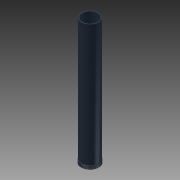
# Autodesk Inventor part: 13_0204_027
Saved by Autodesk Inventor 2012 SP1 (Build 160190100, 190)
## iProperties
Created: 2013-04-03
Part Number: 13_0204_027
Material: Default
Document SubType Name: Modeling
Designer: vogel
Density: 1 g/cm^3
Author: vogel
Autodesk Inventor part; units mm, degrees
ref_plane "YZ Plane" through (0, 0, 0) normal (1, 0, 0) x (0, 1, 0)
ref_plane "XZ Plane" through (0, 0, 0) normal (0, 1, 0) x (-1, 0, 0)
ref_plane "XY Plane" through (0, 0, 0) normal (0, 0, 1) x (1, 0, 0)
sketch "Skizze1" plane through (0, 0, 0) normal (0, 0, 1) x (1, 0, 0)
  circle A0 centre (0, 0) radius 15
  circle A1 centre (0, 0) radius 17.5
  dimension "d0" = 35
  dimension "d1" = 2.5
  constraints: 2 centre point, 2 coincident
  measures "d0" diameter of A1
  measures "d1" radial gap between concentric circles of A1 A0
extrude "Extrusion1" add sketch "Skizze1" along normal blind 250
sketch "Skizze2" plane through (0, 0, 250) normal (0, 0, 1) x (1, 0, 0)
  circle A0 centre (0, 0) radius 17.5 projected
  circle A1 centre (0, 0) radius 17
  dimension "d4" = 34
  constraints: 1 centre point, 1 coincident
  measures "d4" diameter of A1
extrude "Extrusion2" cut sketch "Skizze2" against normal through all
sketch "Skizze3" plane through (0, 0, 0) normal (0, 0, -1) x (-1, 0, 0)
  circle A0 centre (0, 0) radius 17 projected
  circle A1 centre (0, 0) radius 15 projected
  circle A2 centre (0, 0) radius 17.5
  dimension "d7" = 35
  constraints: 1 centre point, 1 coincident
  measures "d7" diameter of A2
extrude "Extrusion3" add sketch "Skizze3" against normal blind 9 contours A2
sketch "Skizze4" plane through (0, 0, 250) normal (0, 0, 1) x (1, 0, 0)
  circle A0 centre (0, 0) radius 17 projected
  circle A1 centre (0, 0) radius 15 projected
  circle A2 centre (0, 0) radius 16.5
  dimension "d10" = 33
  constraints: 1 centre point, 1 coincident
  measures "d10" diameter of A2
extrude "Extrusion4" cut sketch "Skizze4" against normal blind 50 contours A0
sketch "Skizze5" plane through (0, 0, 0) normal (0, 1, 0) x (-1, 0, 0)
  line L0 (-17.5, 9) -> (17.5, 9) projected
  line L1 (17.5, 0) -> (-17.5, 0) projected
  line L2 (17, 9) -> (-17, 9) projected
  line L3 (17.5, 0) -> (17.5, 9) projected
  line L4 (15, 0) -> (15, 250) projected
  line L5 (17, 200) -> (17, 9) projected
  line L6 (17.5, 9) -> (16.75, 9)
  line L7 (16.75, 9) -> (16.75, 7)
  line L8 (16.75, 7) -> (17.5, 7)
  line L9 (17.5, 7) -> (17.5, 9)
  line L10 (24.5, 0) -> (-24.5, 0) projected
  line L11 (0, -50) -> (0, 300) projected
  point P0 (0, 0)
  point P1 (-9.75, 200)
  point P2 (9.75, 200)
  dimension "d13" = 2
  dimension "d14" = 33.5
  constraints: 8 end point, 2 parallel, 1 horizontal, 1 perpendicular, 1 other
  measures "d13" distance of L8.end L3.end
  measures "d14" diameter of L7 L11
revolve "Umdrehung1" cut sketch "Skizze5" angle 360 about axis through (0, 0, -10) along (0, 0, 1) contours L0 L3 L8 L7
chamfer "Fase1" distance 0.75 angle 45 1 edges at (17.5, 0, 7)
thread "Gewinde5" size "M35x1.5" class "6g" standard "ANSI Metric M Profile" full length
sketch "Skizze6" plane through (0, 0, 200) normal (0, 0, 1) x (1, 0, 0)
  circle A0 centre (0, 0) radius 16.5 projected
  circle A1 centre (0, 0) radius 17 projected
extrude "Extrusion5" add sketch "Skizze6" along normal blind 50
